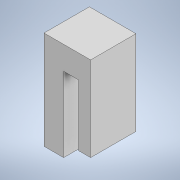
# Autodesk Inventor part: Mount Male
Saved by Autodesk Inventor 2020 (Build 240168000, 168)
## iProperties
Created: 2020-01-14
Part Number: Mount Male
Material: Generic
Document SubType Name: Modeling
Designer: maple
Density: 1 g/cm^3
Appearance: Default
Author: maple
Autodesk Inventor part; units mm, degrees
ref_plane "YZ Plane" through (0, 0, 0) normal (1, 0, 0) x (0, 1, 0)
ref_plane "XZ Plane" through (0, 0, 0) normal (0, 1, 0) x (-1, 0, 0)
ref_plane "XY Plane" through (0, 0, 0) normal (0, 0, 1) x (1, 0, 0)
sketch "Sketch1" plane through (0, 0, 0) normal (0, 1, 0) x (-1, 0, 0)
  line L0 (0, 0) -> (-4.064, 0)
  line L1 (-4.064, 0) -> (-4.064, -9.398)
  line L2 (-4.064, -9.398) -> (0, -9.398)
  line L3 (0, -9.398) -> (0, 0)
  dimension "d0" = 4.064
  dimension "d1" = 9.398
  constraints: 8 end point, 2 parallel, 1 horizontal, 1 perpendicular
  measures "d0" distance of L2.end L1.end
  measures "d1" distance of L1.end L0.end
extrude "Extrusion1" add sketch "Sketch1" along normal blind 20.32
sketch "Sketch3" plane through (4.064, 0, 0) normal (1, 0, 0) x (0, 0, -1)
  line L0 (9.398, 20.32) -> (0, 20.32) projected
  line L1 (9.398, 0) -> (9.398, 20.32) projected
  line L2 (0, 20.32) -> (9.398, 20.32)
  line L3 (9.398, 20.32) -> (9.398, 15.494)
  line L4 (9.398, 15.494) -> (0, 15.494)
  line L5 (0, 15.494) -> (0, 20.32)
  point P0 (0, 0)
  dimension "d5" = 4.826
  constraints: 8 end point, 2 parallel, 1 horizontal, 1 perpendicular, 1 point on line
  measures "d5" distance of L2.end L3.end
extrude "Extrusion2" add sketch "Sketch3" along normal blind 5.588
sketch "Sketch4" plane through (4.064, 15.494, -9.398) normal (0, -1, 0) x (1, 0, 0)
  line L0 (5.588, 0) -> (5.588, 9.398) projected
  line L1 (-4.064, 0) -> (5.588, 0) projected
  line L2 (5.588, 9.398) -> (3.048, 9.398)
  line L3 (3.048, 9.398) -> (3.048, 0)
  line L4 (3.048, 0) -> (5.588, 0)
  line L5 (5.588, 0) -> (5.588, 9.398)
  point P0 (-4.064, 9.398)
  dimension "d8" = 2.54
  constraints: 8 end point, 2 parallel, 1 horizontal, 1 perpendicular, 1 point on line
  measures "d8" distance of L4.end L3.end
extrude "Extrusion3" add sketch "Sketch4" along normal blind 12.7
body "Solid1"
